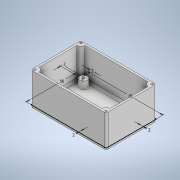
# Autodesk Inventor part: Enclosure
Saved by Autodesk Inventor 2020.2 (Build 242310000, 310)
## iProperties
Created: 2020-09-23
Part Number: Enclosure
Material: Generic
Document SubType Name: Modeling
Designer: johnf
Density: 1 g/cm^3
Appearance: Default
Author: johnf
Autodesk Inventor part; units mm, degrees
ref_plane "YZ Plane" through (0, 0, 0) normal (1, 0, 0) x (0, 1, 0)
ref_plane "XZ Plane" through (0, 0, 0) normal (0, 1, 0) x (-1, 0, 0)
ref_plane "XY Plane" through (0, 0, 0) normal (0, 0, 1) x (1, 0, 0)
sketch "Sketch1" plane through (0, 0, 0) normal (0, 1, 0) x (-1, 0, 0)
  line L0 (26.5, 16.5) -> (-26.5, 16.5) construction
  line L1 (-26.5, 16.5) -> (-26.5, -16.5) construction
  line L2 (-26.5, -16.5) -> (26.5, -16.5) construction
  line L3 (26.5, -16.5) -> (26.5, 16.5) construction
  line L4 (26.5, -16.5) -> (-26.5, 16.5) construction
  circle A0 centre (26.5, 16.5) radius 1
  circle A1 centre (26.5, -16.5) radius 1
  circle A2 centre (-26.5, 16.5) radius 1
  circle A3 centre (-26.5, -16.5) radius 1
  circle A4 centre (26.5, 16.5) radius 3.75
  circle A5 centre (26.5, -16.5) radius 3.75
  circle A6 centre (-26.5, -16.5) radius 3.75
  circle A7 centre (-26.5, 16.5) radius 3.75
  point P0 (0, 0)
  point P1 (0, 0)
  dimension "d0" = 33
  dimension "d1" = 53
  dimension "d2" = 2
  dimension "d3" = 7.5
  constraints: 10 end point, 9 coincident, 8 centre point, 6 equal radius, 2 parallel, 1 horizontal, 1 midpoint, 1 perpendicular
  measures "d0" distance of L2.end L0.start
  measures "d1" distance of L1.end L2.end
  measures "d2" diameter of A0
  measures "d3" diameter of A4
extrude "Extrusion1" add sketch "Sketch1" along normal blind 7.5
sketch "Sketch2" plane through (0, 0, 0) normal (0, 1, 0) x (-1, 0, 0)
  line L0 (37.5, -25) -> (-37.5, -25)
  line L1 (-37.5, -25) -> (-37.5, 25)
  line L2 (-37.5, 25) -> (37.5, 25)
  line L3 (37.5, 25) -> (37.5, -25)
  line L4 (37.5, 25) -> (-37.5, -25) construction
  line L5 (35.5, -19) -> (35.5, 19)
  line L6 (-35.5, 19) -> (-35.5, -19)
  circle A0 centre (-26.5, -16.5) radius 1 projected
  circle A1 centre (26.5, -16.5) radius 3.75 projected
  circle A2 centre (26.5, 16.5) radius 3.75 projected
  circle A3 centre (-26.5, 16.5) radius 3.75 projected
  arc A4 (35.5, -19) -> (31.5, -23) centre (35.5, -23) ccw
  arc A5 (31.5, 23) -> (35.5, 19) centre (35.5, 23) ccw
  arc A6 (-35.5, 19) -> (-31.5, 23) centre (-35.5, 23) ccw
  arc A7 (-31.5, -23) -> (-35.5, -19) centre (-35.5, -23) ccw
  line L7 (-31.5, -23) -> (31.5, -23)
  line L8 (31.5, 23) -> (-31.5, 23)
  point P0 (0, 0)
  point P1 (0, 0)
  dimension "d6" = 75
  dimension "d10" = 50
  dimension "d11" = 2
  dimension "d129" = 4
  dimension "d132" = 2
  dimension "d133" = 2
  dimension "d134" = 2
  constraints: 18 end point, 8 point on circle, 8 point on line, 4 centre point, 4 parallel, 3 equal radius, 2 perpendicular, 1 coincident, 1 horizontal, 1 midpoint
  measures "d6" distance of L0.start L0.end
  measures "d10" distance of L2.end L0.start
  measures "d11" distance between parallel lines of L3 L5
  measures "d129" radius of A4
  measures "d132" distance between parallel lines of L0 L7
  measures "d133" distance between parallel lines of L1 L6
  measures "d134" distance between parallel lines of L2 L8
extrude "Extrusion7" add sketch "Sketch2" against normal blind 2 contours L0 L1 L2 L3 | A4 L7 A7 L6 A6 L8 A5 L5 | A0 | A1 | A2 | A3
extrude "Extrusion8" add sketch "Sketch2" along normal blind 30 contours L0 L1 L2 L3
sketch "Sketch6" plane through (0, 30, 0) normal (0, 1, 0) x (1, 0, 0)
  circle A0 centre (-35.5, 23) radius 1
  line L0 (-32.6716, 23) -> (32.6716, 23) projected
  line L1 (-35.5, -20.1716) -> (-35.5, 20.1716) projected
  circle A1 centre (35.5, 23) radius 1
  circle A2 centre (35.5, -23) radius 1
  circle A3 centre (-35.5, -23) radius 1
  line L2 (35.5, 20.1716) -> (35.5, -20.1716) projected
  line L3 (32.6716, -23) -> (-32.6716, -23) projected
  point P0 (0, 0)
  dimension "d24" = 2
  constraints: 8 point on line, 4 centre point, 3 equal radius
  measures "d24" diameter of A0
extrude "Extrusion9" cut sketch "Sketch6" against normal blind 10
fillet "Fillet2" radius 2 4 edges at (-37.5, 14, -25) (-37.5, 14, 25) (37.5, 14, 25) (37.5, 14, -25)
fillet "Fillet3" radius 2 8 edges at (32.6716, 0, 20.1716) (35.5, 0, 0) (32.6716, 0, -20.1716) (0, 0, -23) (-32.6716, 0, -20.1716) (-35.5, 0, 0) (-32.6716, 0, 20.1716) (0, 0, 23)
body "Solid1"
